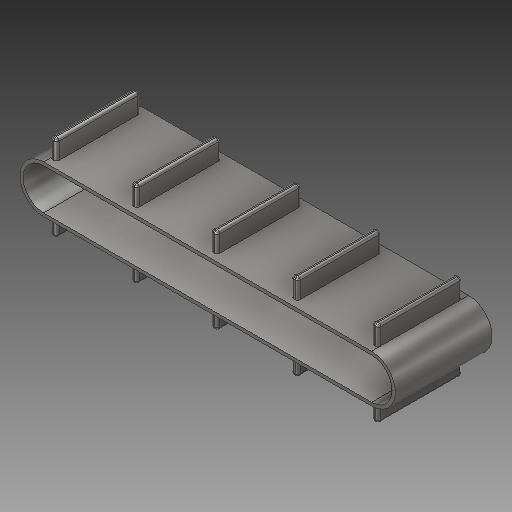
# Autodesk Inventor part: banda
Saved by Autodesk Inventor 2019 (Build 230136000, 136)
## iProperties
Created: 2019-03-24
Part Number: banda
Material: Generic
Document SubType Name: Modeling
Designer: felix
Density: 1 g/cm^3
Appearance: Default
Mass: 1300.09 g
Surface Area: 4588.51 cm^2
Volume: 1300.09 cm^3
Author: felix
Autodesk Inventor part; units mm, degrees
ref_plane "YZ Plane" through (0, 0, 0) normal (1, 0, 0) x (0, 1, 0)
ref_plane "XZ Plane" through (0, 0, 0) normal (0, 1, 0) x (-1, 0, 0)
ref_plane "XY Plane" through (0, 0, 0) normal (0, 0, 1) x (1, 0, 0)
sketch "Sketch1" plane through (0, 0, 0) normal (0, 0, 1) x (1, 0, 0)
  arc A0 (0, 31.75) -> (0, -31.75) centre (0, 0) ccw
  arc A1 (508, -31.75) -> (508, 31.75) centre (508, 0) ccw
  line L0 (508, -31.75) -> (25.9095, -31.75)
  line L1 (0, 31.75) -> (12.9547, 31.75)
  arc A2 (0, 36.75) -> (0, -36.75) centre (0, 0) ccw
  line L2 (0, 36.75) -> (508, 36.75)
  line L3 (508, -36.75) -> (0, -36.75)
  arc A3 (508, -36.75) -> (508, 36.75) centre (508, 0) ccw
  line L4 (495.0453, 31.75) -> (508, 31.75)
  line L5 (12.9547, 31.75) -> (495.0453, 31.75)
  line L6 (25.9095, -31.75) -> (0, -31.75)
  dimension "d0" = 63.5
  dimension "d1" = 508
  dimension "d2" = 73.5
  constraints: 14 end point, 11 tangent, 8 point on circle, 4 centre point, 2 concentric, 2 equal radius, 2 parallel, 1 coincident, 1 horizontal alignment
  measures "d0" diameter of A0
  measures "d1" distance of A1.centre A0.centre
  measures "d2" diameter of A2
extrude "Extrusion1" add sketch "Sketch1" along normal blind 150
sketch "Sketch2" plane through (0, 36.75, 0) normal (0, 1, 0) x (1, 0, 0)
  line L0 (508, 0) -> (508, -150) projected
  line L1 (0, 0) -> (508, 0)
  line L2 (508, 0) -> (508, -10)
  line L3 (508, -10) -> (0, -10)
  line L4 (0, -10) -> (0, 0)
  line L5 (508, -150) -> (0, -150)
  line L6 (0, -140) -> (508, -140)
  line L7 (0, -150) -> (0, -140)
  line L8 (508, -140) -> (508, -150)
  line L9 (0, -10) -> (10, -10)
  line L10 (10, -10) -> (10, -140)
  line L11 (10, -140) -> (0, -140)
  line L12 (0, -140) -> (0, -10)
  line L13 (124.5, -140) -> (124.5, -10)
  line L14 (134.5, -10) -> (134.5, -140)
  line L15 (134.5, -140) -> (124.5, -140)
  line L16 (124.5, -10) -> (134.5, -10)
  line L17 (249, -140) -> (249, -10)
  line L18 (259, -10) -> (259, -140)
  line L19 (259, -140) -> (249, -140)
  line L20 (249, -10) -> (259, -10)
  line L21 (373.5, -140) -> (373.5, -10)
  line L22 (383.5, -10) -> (383.5, -140)
  line L23 (383.5, -140) -> (373.5, -140)
  line L24 (373.5, -10) -> (383.5, -10)
  line L25 (498, -140) -> (498, -10)
  line L26 (508, -10) -> (508, -140)
  line L27 (508, -140) -> (498, -140)
  line L28 (498, -10) -> (508, -10)
  dimension "d5" = 10
  dimension "d8" = 140
  dimension "d13" = 10
  dimension "d16" = 124.5
  constraints: 56 end point, 4 parallel, 3 horizontal, 2 perpendicular, 2 point on line, 1 vertical, 40 other
  measures "d5" distance of L1.end L2.end
  measures "d8" distance of L2.end L5.start
  measures "d13" distance of L10.end L11.end
  measures "d16" distance of L11.end L13.start
extrude "Extrusion2" add sketch "Sketch2" along normal blind 30 contours L0 L6 L25 L3 | L3 L10 L6 L12 | L22 L6 L21 L3 | L3 L14 L6 L13 | L18 L6 L17 L3
fillet "Fillet1" radius 4 40 edges at (0, 66.75, 75) (10, 66.75, 75) (0, 51.75, 10) (10, 51.75, 10) (5, 66.75, 10) (124.5, 66.75, 75) (134.5, 66.75, 75) (124.5, 51.75, 10) (134.5, 51.75, 10) (129.5, 66.75, 10) (249, 66.75, 75) (259, 66.75, 75) (254, 66.75, 10) (249, 51.75, 10) (259, 51.75, 10) (373.5, 66.75, 75) (383.5, 66.75, 75) (378.5, 66.75, 10) (373.5, 51.75, 10) (383.5, 51.75, 10) (498, 66.75, 75) (508, 66.75, 75) (498, 51.75, 10) (508, 51.75, 10) (503, 66.75, 10) (0, 51.75, 140) (5, 66.75, 140) (10, 51.75, 140) (124.5, 51.75, 140) (134.5, 51.75, 140) (129.5, 66.75, 140) (249, 51.75, 140) (259, 51.75, 140) (254, 66.75, 140) (373.5, 51.75, 140) (383.5, 51.75, 140) (378.5, 66.75, 140) (498, 51.75, 140) (508, 51.75, 140) (503, 66.75, 140)
sketch "Sketch4" plane through (0, -36.75, 0) normal (0, -1, 0) x (1, 0, 0)
  line L0 (0, 150) -> (-36.75, 150) projected
  line L1 (508, 136) -> (508, 150) projected
  line L2 (0, 150) -> (508, 150)
  line L3 (508, 150) -> (508, 140)
  line L4 (508, 140) -> (0, 140)
  line L5 (0, 140) -> (0, 150)
  line L6 (0, 10) -> (508, 10)
  line L7 (0, 0) -> (0, 10)
  line L8 (508, 0) -> (0, 0)
  line L9 (508, 10) -> (508, 0)
  line L10 (0, 140) -> (10, 140)
  line L11 (10, 140) -> (10, 10)
  line L12 (10, 10) -> (0, 10)
  line L13 (0, 10) -> (0, 140)
  line L14 (124.5, 10) -> (124.5, 140)
  line L15 (134.5, 140) -> (134.5, 10)
  line L16 (124.5, 140) -> (134.5, 140)
  line L17 (134.5, 10) -> (124.5, 10)
  line L18 (249, 10) -> (249, 140)
  line L19 (259, 140) -> (259, 10)
  line L20 (249, 140) -> (259, 140)
  line L21 (259, 10) -> (249, 10)
  line L22 (373.5, 10) -> (373.5, 140)
  line L23 (383.5, 140) -> (383.5, 10)
  line L24 (373.5, 140) -> (383.5, 140)
  line L25 (383.5, 10) -> (373.5, 10)
  line L26 (498, 10) -> (498, 140)
  line L27 (508, 140) -> (508, 10)
  line L28 (498, 140) -> (508, 140)
  line L29 (508, 10) -> (498, 10)
  point P0 (0, 0)
  dimension "d43" = 10
  dimension "d46" = 140
  dimension "d51" = 10
  dimension "d54" = 124.5
  constraints: 56 end point, 4 parallel, 3 horizontal, 2 perpendicular, 2 point on line, 1 collinear, 1 vertical, 39 other
  measures "d43" distance of L2.end L3.end
  measures "d46" distance of L0.start L6.start
  measures "d51" distance of L11.end L12.end
  measures "d54" distance of L12.end L14.start
extrude "Extrusion4" add sketch "Sketch4" along normal blind 30 contours L27 L6 L26 L4 L1 | L23 L6 L22 L4 | L4 L11 L6 L13 | L19 L6 L18 L4 | L4 L15 L6 L14
fillet "Fillet3" radius 4 40 edges at (5, -66.75, 10) (129.5, -66.75, 10) (254, -66.75, 10) (378.5, -66.75, 10) (503, -66.75, 10) (0, -51.75, 10) (10, -51.75, 10) (124.5, -51.75, 10) (134.5, -51.75, 10) (249, -51.75, 10) (259, -51.75, 10) (373.5, -51.75, 10) (383.5, -51.75, 10) (498, -51.75, 10) (508, -51.75, 10) (0, -51.75, 140) (5, -66.75, 140) (10, -51.75, 140) (124.5, -51.75, 140) (129.5, -66.75, 140) (134.5, -51.75, 140) (249, -51.75, 140) (254, -66.75, 140) (259, -51.75, 140) (378.5, -66.75, 140) (373.5, -51.75, 140) (383.5, -51.75, 140) (498, -51.75, 140) (503, -66.75, 140) (508, -51.75, 140) (0, -66.75, 75) (10, -66.75, 75) (124.5, -66.75, 75) (134.5, -66.75, 75) (249, -66.75, 75) (259, -66.75, 75) (373.5, -66.75, 75) (383.5, -66.75, 75) (498, -66.75, 75) (508, -66.75, 75)
body "Solid1"
